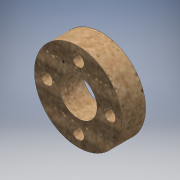
# Autodesk Inventor part: CouplingExtender
Saved by Autodesk Inventor 2016 (Build 200138000, 138)
## iProperties
Created: 2015-11-25
Part Number: CouplingExtender
Material: MDF Medium Density Fiberboard
Document SubType Name: Modeling
Designer: momem
Density: 0.8 g/cm^3
Appearance: Cardboard - Corrugated
Author: momem
Autodesk Inventor part; units mm, degrees
ref_plane "YZ Plane" through (0, 0, 0) normal (1, 0, 0) x (0, 1, 0)
ref_plane "XZ Plane" through (0, 0, 0) normal (0, 1, 0) x (-1, 0, 0)
ref_plane "XY Plane" through (0, 0, 0) normal (0, 0, 1) x (1, 0, 0)
sketch "Sketch1" plane through (0, 0, 0) normal (0, 1, 0) x (-1, 0, 0)
  circle A0 centre (0, 0) radius 11.049
  circle A1 centre (7.9375, 0) radius 1.5
  circle A2 centre (0, 7.9375) radius 1.5
  circle A3 centre (-7.9375, 0) radius 1.5
  circle A4 centre (0, -7.9375) radius 1.5
  circle A5 centre (0, 0) radius 4.7625
  dimension "d0" = 22.098
  dimension "d1" = 3
  dimension "d2" = 7.9375
  dimension "d5" = 360
  dimension "d7" = 9.525
  constraints: 6 centre point, 2 coincident, 1 horizontal alignment, 9 other
  measures "d0" diameter of A0
  measures "d1" diameter of A1
  measures "d2" distance of point (0, 0) A1.centre
  measures "d7" diameter of A5
extrude "Extrusion1" add sketch "Sketch1" along normal blind 5.95
equation "\"d8\" = WoodThickness"
equation "\"WoodThickness\" = 5.95"
body "Solid1"
